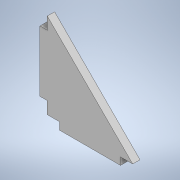
# Autodesk Inventor part: Support Piece
Saved by Autodesk Inventor 2020 (Build 240168000, 168)
## iProperties
Created: 2020-01-30
Part Number: Support Piece
Material: Generic
Document SubType Name: Modeling
Designer: jelte
Density: 1 g/cm^3
Appearance: Default
Mass: 0.78 g
Surface Area: 7.60853 cm^2
Volume: 0.78 cm^3
Author: jelte
Autodesk Inventor part; units mm, degrees
ref_plane "YZ Plane" through (0, 0, 0) normal (1, 0, 0) x (0, 1, 0)
ref_plane "XZ Plane" through (0, 0, 0) normal (0, 1, 0) x (-1, 0, 0)
ref_plane "XY Plane" through (0, 0, 0) normal (0, 0, 1) x (1, 0, 0)
sketch "Sketch1" plane through (0, 0, 0) normal (0, 0, 1) x (1, 0, 0)
  line L0 (-7.2302, -2.2309) -> (-2.2302, -2.2309)
  line L1 (-2.2302, -2.2309) -> (-2.2302, -5.2309)
  line L2 (-2.2302, -5.2309) -> (7.7698, -5.2309)
  line L3 (7.7698, -5.2309) -> (7.7698, -2.2309)
  line L4 (7.7698, -2.2309) -> (12.7698, -2.2309)
  line L5 (-7.2302, -2.2309) -> (-7.2302, 2.7691)
  line L6 (-7.2302, 2.7691) -> (-10.2302, 2.7691)
  line L7 (-10.2302, 2.7691) -> (-10.2302, 12.7691)
  line L8 (-10.2302, 12.7691) -> (-7.2302, 12.7691)
  line L9 (-7.2302, 12.7691) -> (-7.2302, 17.7691)
  line L10 (-7.2302, 17.7691) -> (12.7698, -2.2309)
  point P0 (0, 0)
  dimension "d2" = 5
  dimension "d3" = 5
  dimension "d4" = 10
  dimension "d5" = 5
  dimension "d6" = 10
  dimension "d7" = 5
  constraints: 22 end point, 6 perpendicular, 2 point on line, 2 vertical, 1 horizontal
  measures "d2" distance of L3.end L4.end
  measures "d3" distance of L0.start L0.end
  measures "d4" distance of L1.end L2.end
  measures "d5" distance of L0.start L5.end
  measures "d6" distance of L6.end L7.end
  measures "d7" distance of L8.end L9.end
extrude "Extrusion1" add sketch "Sketch1" along normal blind 3
sketch "Sketch2" plane through (0, 0, 3) normal (0, 0, 1) x (1, 0, 0)
  line L0 (-7.2302, 17.7691) -> (-7.2302, 12.7691) projected
  line L1 (-7.2302, 17.7691) -> (-7.2302, 32.7691)
  line L2 (12.7698, -2.2309) -> (-7.2302, 17.7691) projected
  line L3 (12.7698, -2.2309) -> (27.7698, -2.2309)
  line L4 (-7.2302, 32.7691) -> (27.7698, -2.2309)
  line L5 (-7.2302, 17.7691) -> (12.7698, -2.2309)
  point P0 (0, 0)
  dimension "d14" = 15
  dimension "d15" = 15
  constraints: 8 end point, 1 collinear, 1 horizontal, 1 vertical
  measures "d14" distance of L0.start L1.end
  measures "d15" distance of L2.start L3.end
extrude "Extrusion2" add sketch "Sketch2" against normal blind 3
sketch "Sketch3" plane through (-10.2302, 12.7691, 0) normal (0, 1, 0) x (1, 0, 0)
  line L0 (0, 0) -> (0, -3) projected
  line L1 (3, 0) -> (3, -3) projected
  line L2 (0, 0) -> (3, 0)
  line L3 (3, 0) -> (3, -3)
  line L4 (3, -3) -> (0, -3)
  line L5 (0, -3) -> (0, 0)
  point P0 (10.2302, 0)
  constraints: 8 end point, 2 parallel, 1 horizontal, 1 perpendicular
extrude "Extrusion3" add sketch "Sketch3" along normal blind 15
sketch "Sketch4" plane through (7.7698, -5.2309, 0) normal (1, 0, 0) x (0, 0, -1)
  line L0 (-3, 3) -> (-3, 0) projected
  line L1 (-3, 3) -> (0, 3)
  line L2 (0, 3) -> (0, 0)
  line L3 (0, 0) -> (-3, 0)
  line L4 (-3, 0) -> (-3, 3)
  point P0 (0, 5.2309)
  constraints: 8 end point, 2 parallel, 1 horizontal, 1 perpendicular
extrude "Extrusion4" add sketch "Sketch4" along normal blind 15
body "Solid1"
